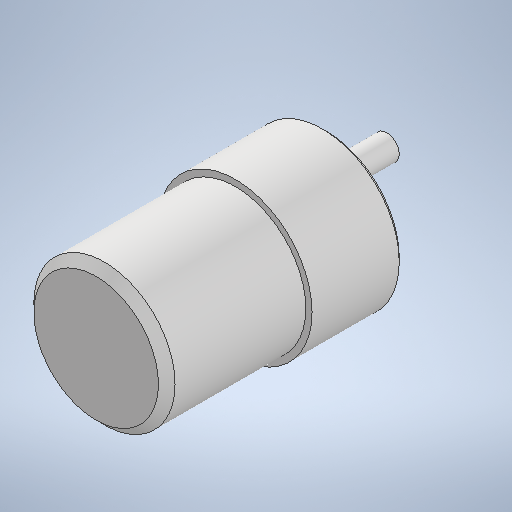
# Autodesk Inventor part: JGB37-520
Saved by Autodesk Inventor 2025.1 (Build 291241000, 241)
## iProperties
Created: 2025-08-26
Part Number: JGB37-520
Material: 常规
Document SubType Name: Modeling
Designer: Piw
Density: 1 g/cm^3
Appearance: 默认
Author: Piw
Autodesk Inventor part; units mm, degrees
ref_plane "YZ Plane" through (0, 0, 0) normal (1, 0, 0) x (0, 1, 0)
ref_plane "XZ Plane" through (0, 0, 0) normal (0, 1, 0) x (-1, 0, 0)
ref_plane "XY Plane" through (0, 0, 0) normal (0, 0, 1) x (1, 0, 0)
sketch "草图1" plane through (0, 0, 0) normal (0, 0, 1) x (1, 0, 0)
  circle A0 centre (0, 0) radius 18.5
  dimension "d0" = 37
  constraints: 1 centre point, 1 coincident
  measures "d0" diameter of A0
extrude "拉伸1" add sketch "草图1" along normal blind 22
sketch "草图2" plane through (0, 0, 22) normal (0, 0, 1) x (1, 0, 0)
  circle A0 centre (0, 0) radius 17
  dimension "d3" = 34
  constraints: 1 centre point, 1 coincident
  measures "d3" diameter of A0
extrude "拉伸2" add sketch "草图2" along normal blind 33.5
chamfer "倒角1" distance 2 angle 45 1 edges at (-17, 0, 55.5)
sketch "草图3" plane through (0, 0, 0) normal (0, 0, -1) x (-1, 0, 0)
  circle A0 centre (7, 0) radius 5
  line L0 (33.5538, 0) -> (-37.1398, 0)
  point P0 (0, 0)
  dimension "d9" = 10
  dimension "d10" = 7
  constraints: 2 end point, 2 horizontal, 1 centre point, 1 point on line
  measures "d9" diameter of A0
  measures "d10" distance of point (0, 0) A0.centre
extrude "拉伸3" add sketch "草图3" along normal blind 6
sketch "草图4" plane through (-7, 0, -6) normal (0, 0, -1) x (-1, 0, 0)
  circle A0 centre (0, 0) radius 5 projected
  circle A1 centre (0, 0) radius 3
  point P0 (-7, 0)
  dimension "d13" = 6
  constraints: 1 centre point, 1 coincident
  measures "d13" diameter of A1
extrude "拉伸4" add sketch "草图4" along normal blind 15.5 contours A1
chamfer "倒角2" distance 0.5 angle 45 1 edges at (-2, 0, -6)
sketch "草图5" plane through (0, 0, 0) normal (0, 0, -1) x (-1, 0, 0)
  circle A0 centre (7, 0) radius 5 projected
  circle A1 centre (7, 0) radius 7
  circle A2 centre (0, 0) radius 11
  point P0 (8.6429, -6.8045)
  point P1 (8.6429, 6.8045)
  dimension "d19" = 22
  constraints: 1 centre point, 1 coincident, 3 other
  measures "d19" diameter of A2
extrude "拉伸5" cut sketch "草图5" against normal blind 1 contours A1 A2
chamfer "倒角3" distance 1 angle 45 2 edges at (11, 0, 0) (-18.5, 0, 0)
